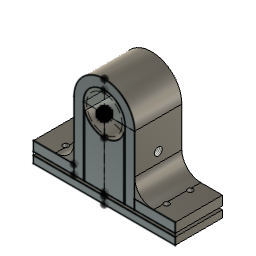
floorcowl_bottomfloor v13 (Autodesk Fusion 360 design; units mm, degrees)
Autodesk Fusion 360 part; units mm, degrees
sketch "Sketch1" plane through (0, 0, 0) normal (0, 1, 0) x (1, 0, 0)
  circle A0 centre (0, 0) radius 9.525 construction
  circle A1 centre (0, 0) radius 11.176 construction
  line L0 (0, 0) -> (0, 36.576)
  line L1 (0, 36.576) -> (38.1, 36.576) construction
  line L2 (38.1, 36.576) -> (38.1, 38.3286) construction
  line L3 (38.1, 38.3286) -> (0, 38.3286) construction
  line L4 (0, 38.3286) -> (0, 36.576) construction
  line L5 (0, 36.576) -> (-38.1, 36.576) construction
  line L6 (-38.1, 38.3286) -> (0, 38.3286) construction
  line L7 (-38.1, 36.576) -> (-38.1, 38.3286) construction
  line L8 (0, 38.3286) -> (38.1, 38.3286)
  line L9 (38.1, 38.3286) -> (38.1, 42.1386)
  line L10 (38.1, 42.1386) -> (0, 42.1386)
  line L11 (0, 42.1386) -> (0, 38.3286)
  line L12 (-38.1, 42.1386) -> (0, 42.1386)
  line L13 (0, 38.3286) -> (-38.1, 38.3286)
  line L14 (-38.1, 38.3286) -> (-38.1, 42.1386)
  line L15 (0, 0) -> (11.176, 0)
  line L16 (0, 0) -> (-11.176, 0)
  line L17 (11.176, 0) -> (16.256, 0) construction
  line L18 (16.256, 0) -> (16.256, 36.576)
  line L19 (16.256, 36.576) -> (11.176, 36.576)
  line L20 (11.176, 36.576) -> (11.176, 0)
  arc A2 (0, -16.256) -> (16.256, 0) centre (0, 0) ccw
  line L21 (0, 0) -> (0, -16.256) construction
  line L22 (0, 0) -> (16.256, 0) construction
  arc A3 (0, -11.176) -> (11.176, 0) centre (0, 0) ccw
  arc A4 (-16.256, 0) -> (0, -16.256) centre (0, 0) ccw
  arc A5 (-11.176, 0) -> (0, -11.176) centre (0, 0) ccw
  line L23 (-16.256, 0) -> (-16.256, 36.576)
  line L24 (-11.176, 36.576) -> (-11.176, 0)
  line L25 (-16.256, 36.576) -> (-11.176, 36.576)
  line L26 (0, 11.176) -> (0, 36.576)
  arc A6 (10.502, 3.8224) -> (0, 11.176) centre (0, 0) ccw
  line L27 (0, 0) -> (10.502, 3.8224) construction
  line L28 (0, 0) -> (0, 11.176) construction
  line L29 (10.502, 3.8224) -> (10.502, 36.576)
  line L30 (10.502, 36.576) -> (0, 36.576)
  arc A7 (0, 11.176) -> (-10.502, 3.8224) centre (0, 0) ccw
  line L31 (-10.502, 3.8224) -> (-10.502, 36.576)
  line L32 (-10.502, 36.576) -> (0, 36.576)
  line L33 (16.256, 36.576) -> (38.1, 36.576)
  line L34 (38.1, 36.576) -> (38.1, 31.496)
  line L35 (38.1, 31.496) -> (16.256, 31.496)
  line L36 (16.256, 31.496) -> (16.256, 36.576)
  line L37 (-38.1, 31.496) -> (-16.256, 31.496)
  line L38 (-38.1, 36.576) -> (-38.1, 31.496)
  line L39 (-16.256, 36.576) -> (-38.1, 36.576)
  dimension "d1" = 19.05
  dimension "d2" = 22.352
  dimension "d3" = 36.576
  dimension "d4" = 38.1
  dimension "d5" = 1.7526
  dimension "d6" = 38.1
  dimension "d7" = 3.81
  dimension "d8" = 5.08
  dimension "d9" = 36.576
  dimension "d10" = 90
  dimension "d11" = 70
  dimension "d12" = 5.08
  dimension "d13" = 21.844
  constraint coincident A0.centre A1.centre
  constraint concentric A0 A1
  constraint vertical L0
  constraint horizontal L1
  constraint vertical L2
  constraint horizontal L3
  constraint vertical L4
  constraint symmetric L0.end L4 L1.start
  constraint symmetric L1.end L4 L5.end
  constraint symmetric L2.end L4 L6.start
  constraint symmetric L3.end L4 L6.end
  constraint horizontal L8
  constraint vertical L9
  constraint horizontal L10
  constraint vertical L11
  constraint symmetric L3.end L11 L4.start
  constraint symmetric L2.end L11 L6.start
  constraint symmetric L9.end L11 L12.start
  constraint symmetric L10.end L11 L12.end
  constraint coincident A1 L15.end
  constraint perpendicular L0 L15
  constraint coincident A1 L16.end
  constraint parallel L15 L16
  constraint horizontal L17
  constraint vertical L18
  constraint horizontal L19
  constraint vertical L20
  constraint coincident L21 A3.start
  constraint symmetric L0 L15.end L16.end
  constraint symmetric L0 L17.end A4.start
  constraint symmetric L0 L18.end L23.end
  constraint symmetric L0 L19.end L24.start
  constraint symmetric L0 A2.start L21.end
  constraint symmetric L0 A2 A4
  constraint symmetric L0 A3.start A5.end
  constraint symmetric L0 A3 A5
  constraint coincident A1 L26.start
  constraint coincident L0 L26.start
  constraint coincident L1 L29.end
  constraint perpendicular L1 L29
  constraint symmetric L0 L1.start L4.end
  constraint symmetric L0 L26.start A6.end
  constraint symmetric L0 A6.start A7.end
  constraint symmetric L0 A6 A7
  constraint symmetric L0 L29.end L31.end
  constraint horizontal L33
  constraint vertical L34
  constraint horizontal L35
  constraint vertical L36
  constraint symmetric L0 L1.end L5.end
  constraint symmetric L0 L34.end L37.start
  constraint symmetric L0 L35.end L37.end
  measures "d1" diameter of A0
  measures "d2" diameter of A1
  measures "d3" distance of A0.centre L0.end
  measures "d4" distance of L0.end L1.end
  measures "d5" distance of L0.end L3.end
  measures "d6" distance of L3.end L2.end
  measures "d7" distance of L3.end L10.end
  measures "d8" distance of L15.end L17.end
  measures "d9" distance of L15.end L19.end
  measures "d10" angle of L21 L22
  measures "d11" angle of L27 L28
  measures "d12" distance of L18.end L35.end
  measures "d13" distance of L34.end L35.end
extrude "Extrude1" add sketch "Sketch1" along normal blind 25.4 contours L8 L9 L10 L11 | L11 L12 L13 L14 | L18 L19 L20 A2 A3 A4 A5 L23 L24 L25 L36 | L18 L33 L34 L35 L36 | L23 L37 L38 L39 makes body 1 at (-16.1752, 16.9333, 1.6186) makes body 2 at (12.7, 8.4667, -42.1386)
extrude "Extrude2" add sketch "Sketch1" along normal blind 25.4 separate body contours L0 L26 A7 L31 L32 | L0 L26 A6 L29 L30 makes body 3
sketch "Sketch3" plane through (16.256, 0, 0) normal (1, 0, 0) x (0, 1, 0)
  line L0 (0, 0) -> (0, -31.496)
  line L1 (0, -31.496) -> (25.4, -31.496)
  line L2 (25.4, -31.496) -> (25.4, 0)
  line L3 (25.4, 0) -> (0, 0)
  line L4 (25.4, 0) -> (0, 0) construction
  line L5 (0, 0) -> (0, -31.496) construction
  line L6 (0, -31.496) -> (25.4, -31.496) construction
  line L7 (25.4, -31.496) -> (25.4, 0) construction
  line L8 (12.7, 0) -> (12.7, -31.496) construction
  line L9 (0, -15.748) -> (25.4, -15.748) construction
  point P0 (12.7, -15.748)
  constraint horizontal L4
  constraint vertical L5
  constraint horizontal L6
  constraint vertical L7
  constraint coincident L0.end L1.start
  constraint coincident L2.end L3.start
  constraint midpoint L4 L8.start
  constraint midpoint L6 L8.end
  constraint midpoint L5 L9.start
  constraint midpoint L7 L9.end
  constraint midpoint L9 P0
sketch "Sketch5" plane through (0, 0, -42.1386) normal (0, 0, -1) x (1, 0, 0)
  line L0 (38.1, 0) -> (-38.1, 0)
  line L1 (-38.1, 0) -> (-38.1, -25.4)
  line L2 (-38.1, -25.4) -> (38.1, -25.4)
  line L3 (38.1, -25.4) -> (38.1, 0)
  line L4 (-38.1, -25.4) -> (-16.256, -25.4)
  line L5 (-16.256, -25.4) -> (-16.256, 0)
  line L6 (-16.256, 0) -> (-38.1, 0)
  line L7 (-38.1, 0) -> (-38.1, -25.4)
  line L8 (0, 0) -> (0, -25.4)
  line L9 (-27.178, -25.4) -> (-27.178, 0)
  line L10 (-16.256, -12.7) -> (-38.1, -12.7)
  point P0 (-27.178, -19.05)
  point P1 (-27.178, -6.35)
  point P2 (27.178, -19.05)
  point P3 (27.178, -6.35)
  dimension "d30" = 21.844
  dimension "d31" = 25.4
  dimension "d32" = 6.35
  constraint horizontal L4
  constraint vertical L5
  constraint horizontal L6
  constraint vertical L7
  constraint coincident L1.end L2.start
  constraint coincident L8.start origin
  constraint midpoint L2 L8.end
  constraint midpoint L4 L9.start
  constraint midpoint L6 L9.end
  constraint midpoint L5 L10.start
  constraint midpoint L7 L10.end
  constraint coincident L9 P0
  constraint symmetric L10 P0 P1
  constraint symmetric L8 P0 P2
  constraint symmetric L8 P1 P3
  measures "d30" distance of L1.end L4.end
  measures "d31" distance of L1.end L0.end
  measures "d32" distance of L4 P0
hole "Hole3" at (27.178, 19.05, -42.1386) at (27.178, 6.35, -42.1386) at (-27.178, 19.05, -42.1386) at (-27.178, 6.35, -42.1386) direction (0, 0, 1) diameter 2.8702 depth 11.1125 tip angle 180 bodies 1 2
hole "Hole4" at (16.256, 12.7, -15.748) direction (-1, 0, 0) diameter 4.2418 depth 30 tip angle 180 bodies 1 3
thread "Thread4" "ISO Metric profile 5.0 M5x0.8 M5x0.8 6H" thread offset 0 thread depth 5.9436
fillet "Fillet1" radius 10.16 2 edges at (-16.256, 12.7, -31.496) (16.256, 12.7, -31.496) on bodies 1
equation "d33 = ( 7 / 16 ) * 1 in"
